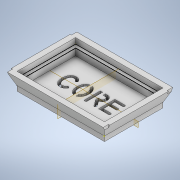
# Autodesk Inventor part: Rack holder Kinpen V2
Saved by Autodesk Inventor 2022 (Build 260153000, 153)
## iProperties
Created: 2021-05-21
Part Number: Rack holder Kinpen V2
Material: Generic
Document SubType Name: Modeling
Designer: Olivi
Density: 1 g/cm^3
Appearance: Default
Author: Olivi
Autodesk Inventor part; units mm, degrees
ref_plane "YZ Plane" through (0, 0, 0) normal (1, 0, 0) x (0, 1, 0)
ref_plane "XZ Plane" through (0, 0, 0) normal (0, 1, 0) x (-1, 0, 0)
ref_plane "XY Plane" through (0, 0, 0) normal (0, 0, 1) x (1, 0, 0)
sketch "Sketch1" plane through (0, 0, 0) normal (0, 1, 0) x (-1, 0, 0)
  line L0 (0, 0) -> (0, -85.5)
  line L1 (0, -85.5) -> (127.8, -85.5)
  line L2 (127.8, -85.5) -> (127.8, 0)
  line L3 (127.8, 0) -> (0, 0)
  dimension "d0" = 85.5
  dimension "d1" = 127.8
  constraints: 8 end point, 3 perpendicular, 1 vertical
  measures "d0" distance of L0.start L0.end
  measures "d1" distance of L0.end L1.end
extrude "Extrusion2" add sketch "Sketch1" along normal blind 7
sketch "Sketch3" plane through (0, 7, 0) normal (0, 1, 0) x (1, 0, 0)
  point P0 (0, 0)
sketch "Sketch5" plane through (0, 7, 0) normal (0, 1, 0) x (1, 0, 0)
  line L0 (-127.8, 0) -> (0, 0) projected
  line L1 (-127.8, 0) -> (0, 0)
  line L2 (0, 0) -> (0, 85.5) projected
  line L3 (0, 0) -> (0, 85.5)
  line L4 (0, 85.5) -> (-127.8, 85.5) projected
  line L5 (0, 85.5) -> (-127.8, 85.5)
  line L6 (-127.8, 85.5) -> (-127.8, 0)
  line L7 (-122.8, 80.5) -> (-5, 80.5)
  line L8 (-5, 80.5) -> (-5, 4.1226)
  line L9 (-5, 4.1226) -> (-122.8, 4.1226)
  line L10 (-122.8, 4.1226) -> (-122.8, 80.5)
  line L11 (-127.8, 85.5) -> (-127.8, 0) projected
  dimension "d44" = 5
  dimension "d45" = 5
  dimension "d46" = 5
  constraints: 16 end point, 5 perpendicular, 3 equal length
  measures "d44" distance between parallel lines of L2 L8
  measures "d45" distance between parallel lines of L6 L10
  measures "d46" distance between parallel lines of L4 L7
extrude "Extrusion4" add sketch "Sketch5" along normal blind 10
sketch "Sketch9" plane through (0, 17, 0) normal (0, 1, 0) x (1, 0, 0)
  line L0 (-127.8, 85.5) -> (-127.8, 0) projected
  line L1 (-127.8, 0) -> (-127.8, 85.5)
  line L2 (-127.8, 85.5) -> (0, 85.5)
  line L3 (0, 85.5) -> (0, 0)
  line L4 (0, 0) -> (-127.8, 0)
  line L5 (-122.8, 4.1226) -> (-5, 4.1226) projected
  line L6 (-5, 80.5) -> (-122.8, 80.5) projected
  line L7 (-122.8, 4.1226) -> (-122.8, 80.5)
  line L8 (-122.8, 80.5) -> (-5, 80.5)
  line L9 (-5, 80.5) -> (-5, 4.1226)
  line L10 (-5, 4.1226) -> (-122.8, 4.1226)
  point P0 (0, 0)
  constraints: 16 end point, 5 equal length, 3 perpendicular
ref_plane "Work Plane4" through (-63.9, 0, 0) normal (1, 0, 0) x (0, 0, -1)
sketch "Sketch21" plane through (-63.9, 0, 0) normal (1, 0, 0) x (0, 0, -1)
  line L0 (0, 0) -> (0, 17) projected
  line L1 (0, 7.0438) -> (0, 25.0438)
  line L2 (0, 25.0438) -> (-8, 25.0438)
  line L3 (-8, 25.0438) -> (0, 7.0438)
  line L4 (85.5, 0) -> (85.5, 17) projected
  line L5 (85.5, 7.0438) -> (85.5, 25.0438)
  line L6 (85.5, 25.0438) -> (93.5, 25.0438)
  line L7 (93.5, 25.0438) -> (85.5, 7.0438)
  dimension "d99" = 18
  dimension "d100" = 8
  dimension "d101" = 18
  dimension "d102" = 8
  constraints: 12 end point, 2 collinear, 2 perpendicular, 2 point on line
  measures "d99" distance of L1.start L1.end
  measures "d100" distance of L1.end L2.end
  measures "d101" distance of L5.start L5.end
  measures "d102" distance of L5.end L6.end
extrude "Extrusion7" add sketch "Sketch21" along normal mid plane 140
ref_plane "Work Plane5" through (-127.8, 0, -42.7) normal (0, 0, 1) x (1, 0, 0)
sketch "Sketch22" plane through (-127.8, 0, -42.7) normal (0, 0, 1) x (1, 0, 0)
  line L0 (127.8, 7.0438) -> (133.9, 7.0438) projected
  line L1 (127.8, 7.0438) -> (127.8, 25.0438)
  line L2 (133.9, 25.0438) -> (-6.1, 25.0438) projected
  line L3 (127.8, 25.0438) -> (135.8, 25.0438)
  line L4 (135.8, 25.0438) -> (127.8, 7.0438)
  line L5 (0, 0) -> (0, 7.0438) projected
  line L6 (0, 7.0438) -> (0, 25.0438)
  line L7 (0, 25.0438) -> (-8, 25.0438)
  line L8 (-6.1, 7.0438) -> (0, 7.0438) projected
  line L9 (-8, 25.0438) -> (0, 7.0438)
  point P0 (127.8, 0)
  dimension "d106" = 8
  dimension "d107" = 8
  constraints: 12 end point, 3 point on line, 2 perpendicular, 1 vertical
  measures "d106" distance of L1.end L3.end
  measures "d107" distance of L6.end L7.end
extrude "Extrusion8" add sketch "Sketch22" along normal mid plane 86
sketch "Sketch24" plane through (-127.8, 0, 0) normal (0, 0, 1) x (1, 0, 0)
  line L0 (-6.1, 7.0438) -> (-6.1, 25.0438) projected
  line L1 (0, 7.0438) -> (127.8, 7.0438) projected
  line L2 (-6.1, 20.9849) -> (0, 7.0438)
  line L3 (0, 7.0438) -> (-6.1, 7.0438)
  line L4 (-6.1, 7.0438) -> (-6.1, 20.9849)
  line L5 (127.8, 7.0438) -> (133.9, 7.0438) projected
  line L6 (133.9, 7.0438) -> (133.9, 20.7688) projected
  line L7 (127.8, 7.0438) -> (133.9, 20.7688)
  line L8 (133.9, 20.7688) -> (133.9, 7.0438)
  line L9 (133.9, 7.0438) -> (127.8, 7.0438)
  point P0 (127.8, 0)
  constraints: 12 end point, 2 collinear, 2 perpendicular, 1 point on line
extrude "Extrusion9" cut sketch "Sketch24" along normal blind 86
sketch "Sketch25" plane through (0, 0, -85.5) normal (0, 0, -1) x (-1, 0, 0)
  line L0 (-6.1, 20.7688) -> (0, 7.0438) projected
  line L1 (0, 7.0438) -> (-6.1, 20.7688)
  line L2 (-6.1, 20.7688) -> (-6.1, 7.0438)
  line L3 (-6.1, 7.0438) -> (0, 7.0438)
  line L4 (127.8, 7.0438) -> (133.9, 20.7688) projected
  line L5 (127.8, 7.0438) -> (133.9, 20.7688)
  line L6 (133.9, 7.0438) -> (133.9, 20.7688) projected
  line L7 (133.9, 20.7688) -> (133.9, 7.0438)
  line L8 (127.8, 7.0438) -> (0, 7.0438) projected
  line L9 (133.9, 7.0438) -> (127.8, 7.0438)
  point P0 (0, 0)
  constraints: 12 end point, 3 collinear, 2 perpendicular, 1 point on line, 1 vertical
extrude "Extrusion10" cut sketch "Sketch25" along normal blind 86
sketch "Sketch26" plane through (0, 7, 0) normal (0, 1, 0) x (1, 0, 0)
  line L0 (-106.3, 54.404) -> (-23.0142, 54.404) construction
  line L1 (-23.0142, 54.404) -> (-23.0142, 29.6305) construction
  line L2 (-23.0142, 29.6305) -> (-106.3, 29.6305) construction
  line L3 (-106.3, 29.6305) -> (-106.3, 54.404) construction
  line L4 (-122.8, 80.5) -> (-5, 80.5) projected
  line L5 (-5, 4.1226) -> (-122.8, 4.1226) projected
  line L6 (-122.8, 4.1226) -> (-122.8, 80.5) projected
  spline S0 degree 2 poles (-87.6379, 33.5693) (-89.4205, 31.3781) (-92.8187, 29.6883) (-95.2142, 29.6883) knots 0 0 0 1 2 2 2
  spline S1 degree 2 poles (-95.2142, 29.6883) (-99.2994, 29.6883) (-101.8805, 33.1422) knots 0 0 0 1 1 1
  spline S2 degree 2 poles (-101.8805, 33.1422) (-104.5359, 36.6332) (-104.5359, 42.2783) knots 0 0 0 1 1 1
  spline S3 degree 2 poles (-104.5359, 42.2783) (-104.5359, 48.5175) (-101.5463, 51.7857) knots 0 0 0 1 1 1
  spline S4 degree 2 poles (-101.5463, 51.7857) (-99.1508, 54.404) (-95.697, 54.404) knots 0 0 0 1 1 1
  spline S5 degree 2 poles (-95.697, 54.404) (-93.0044, 54.404) (-91.4446, 53.6055) knots 0 0 0 1 1 1
  spline S6 degree 2 poles (-91.4446, 53.6055) (-89.7177, 52.7142) (-88.5107, 50.5045) knots 0 0 0 1 1 1
  spline S7 degree 2 poles (-88.5107, 50.5045) (-88.2507, 50.0402) (-88.2507, 49.6131) knots 0 0 0 1 1 1
  spline S8 degree 2 poles (-88.2507, 49.6131) (-88.2507, 48.8704) (-89.3648, 47.8491) (-90.0519, 47.8491) knots 0 0 0 1 2 2 2
  spline S9 degree 2 poles (-90.0519, 47.8491) (-91.0175, 47.8491) (-91.5746, 48.8889) knots 0 0 0 1 1 1
  spline S10 degree 2 poles (-91.5746, 48.8889) (-92.2059, 49.9659) (-93.283, 50.4302) knots 0 0 0 1 1 1
  spline S11 degree 2 poles (-93.283, 50.4302) (-94.1, 50.8201) (-95.7155, 50.8201) knots 0 0 0 1 1 1
  spline S12 degree 2 poles (-95.7155, 50.8201) (-97.8139, 50.8201) (-99.2623, 48.9446) knots 0 0 0 1 1 1
  spline S13 degree 2 poles (-99.2623, 48.9446) (-101.0449, 46.6792) (-101.0449, 42.2783) knots 0 0 0 1 1 1
  spline S14 degree 2 poles (-101.0449, 42.2783) (-101.0449, 38.2302) (-97.6839, 33.2722) (-95.1584, 33.2722) knots 0 0 0 1 2 2 2
  spline S15 degree 2 poles (-95.1584, 33.2722) (-92.4288, 33.2722) (-90.3676, 35.8719) knots 0 0 0 1 1 1
  spline S16 degree 2 poles (-90.3676, 35.8719) (-89.8476, 36.5032) (-89.0492, 36.5032) knots 0 0 0 1 1 1
  spline S17 degree 2 poles (-89.0492, 36.5032) (-88.3621, 36.5032) (-87.2108, 35.4077) (-87.2108, 34.6835) knots 0 0 0 1 2 2 2
  spline S18 degree 2 poles (-87.2108, 34.6835) (-87.2108, 34.0892) (-87.6379, 33.5693) knots 0 0 0 1 1 1
  spline S19 degree 2 poles (-64.3335, 41.944) (-64.3335, 37.0417) (-66.6361, 33.8478) knots 0 0 0 1 1 1
  spline S20 degree 2 poles (-66.6361, 33.8478) (-69.3286, 29.6883) (-73.4696, 29.6883) knots 0 0 0 1 1 1
  spline S21 degree 2 poles (-73.4696, 29.6883) (-77.6291, 29.6883) (-80.2845, 33.5322) knots 0 0 0 1 1 1
  spline S22 degree 2 poles (-80.2845, 33.5322) (-82.7542, 37.0603) (-82.7542, 41.944) knots 0 0 0 1 1 1
  spline S23 degree 2 poles (-82.7542, 41.944) (-82.7542, 46.8277) (-80.433, 50.4116) knots 0 0 0 1 1 1
  spline S24 degree 2 poles (-80.433, 50.4116) (-77.8705, 54.404) (-73.8595, 54.404) knots 0 0 0 1 1 1
  spline S25 degree 2 poles (-73.8595, 54.404) (-69.57, 54.404) (-66.8032, 50.4302) knots 0 0 0 1 1 1
  spline S26 degree 2 poles (-66.8032, 50.4302) (-64.3335, 46.8277) (-64.3335, 41.944) knots 0 0 0 1 1 1
  spline S27 degree 2 poles (-67.8616, 41.944) (-67.8616, 45.5093) (-69.4215, 48.1833) knots 0 0 0 1 1 1
  spline S28 degree 2 poles (-69.4215, 48.1833) (-71.0556, 50.8201) (-73.8595, 50.8201) knots 0 0 0 1 1 1
  spline S29 degree 2 poles (-73.8595, 50.8201) (-76.4406, 50.8201) (-78.0376, 47.8862) knots 0 0 0 1 1 1
  spline S30 degree 2 poles (-78.0376, 47.8862) (-79.226, 45.6022) (-79.226, 41.944) knots 0 0 0 1 1 1
  spline S31 degree 2 poles (-79.226, 41.944) (-79.226, 38.3602) (-78.1304, 36.1133) knots 0 0 0 1 1 1
  spline S32 degree 2 poles (-78.1304, 36.1133) (-76.1807, 33.2722) (-73.4696, 33.2722) knots 0 0 0 1 1 1
  spline S33 degree 2 poles (-73.4696, 33.2722) (-70.7956, 33.2722) (-69.1244, 36.1133) knots 0 0 0 1 1 1
  spline S34 degree 2 poles (-69.1244, 36.1133) (-67.8616, 38.323) (-67.8616, 41.944) knots 0 0 0 1 1 1
  spline S35 degree 2 poles (-42.9417, 47.032) (-42.9417, 43.281) (-45.9871, 41.2941) knots 0 0 0 1 1 1
  spline S36 degree 2 poles (-45.9871, 41.2941) (-47.0641, 40.1242) (-48.7353, 40.1242) knots 0 0 0 1 1 1
  line L7 (-48.7353, 40.1242) -> (-43.2945, 32.7708)
  spline S37 degree 2 poles (-43.2945, 32.7708) (-42.9417, 32.2323) (-42.9417, 31.6938) knots 0 0 0 1 1 1
  spline S38 degree 2 poles (-42.9417, 31.6938) (-42.9417, 30.951) (-44.0373, 29.8554) (-44.7429, 29.8554) knots 0 0 0 1 2 2 2
  spline S39 degree 2 poles (-44.7429, 29.8554) (-45.5785, 29.8554) (-46.117, 30.6725) knots 0 0 0 1 1 1
  line L8 (-46.117, 30.6725) -> (-52.7834, 40.1242)
  line L9 (-52.7834, 40.1242) -> (-56.7572, 40.1242)
  line L10 (-56.7572, 40.1242) -> (-56.7572, 31.6938)
  spline S40 degree 2 poles (-56.7572, 31.6938) (-56.7572, 29.8554) (-58.5213, 29.8554) knots 0 0 0 1 1 1
  spline S41 degree 2 poles (-58.5213, 29.8554) (-60.2854, 29.8554) (-60.2854, 31.6938) knots 0 0 0 1 1 1
  line L11 (-60.2854, 31.6938) -> (-60.2854, 54.1626)
  line L12 (-60.2854, 54.1626) -> (-49.9795, 54.1626)
  spline S42 degree 2 poles (-49.9795, 54.1626) (-47.1198, 54.1626) (-45.0957, 52.3242) knots 0 0 0 1 1 1
  spline S43 degree 2 poles (-45.0957, 52.3242) (-42.9417, 50.2816) (-42.9417, 47.032) knots 0 0 0 1 1 1
  spline S44 degree 2 poles (-46.4327, 47.032) (-46.4327, 48.7032) (-47.3426, 49.6131) knots 0 0 0 1 1 1
  spline S45 degree 2 poles (-47.3426, 49.6131) (-48.4939, 50.6159) (-49.9795, 50.6159) knots 0 0 0 1 1 1
  line L13 (-49.9795, 50.6159) -> (-56.7572, 50.6159)
  line L14 (-56.7572, 50.6159) -> (-56.7572, 43.7081)
  line L15 (-56.7572, 43.7081) -> (-48.7353, 43.7081)
  spline S46 degree 2 poles (-48.7353, 43.7081) (-48.1225, 43.7081) (-47.4169, 44.3395) knots 0 0 0 1 1 1
  spline S47 degree 2 poles (-47.4169, 44.3395) (-46.4327, 45.2494) (-46.4327, 47.032) knots 0 0 0 1 1 1
  line L16 (-24.4467, 30.1711) -> (-38.8936, 30.1711)
  line L17 (-38.8936, 30.1711) -> (-38.8936, 54.1812)
  line L18 (-38.8936, 54.1812) -> (-24.4467, 54.1812)
  spline S48 degree 2 poles (-24.4467, 54.1812) (-22.6826, 54.1812) (-22.6826, 52.3985) knots 0 0 0 1 1 1
  spline S49 degree 2 poles (-22.6826, 52.3985) (-22.6826, 50.5973) (-24.4467, 50.5973) knots 0 0 0 1 1 1
  line L19 (-24.4467, 50.5973) -> (-35.4026, 50.5973)
  line L20 (-35.4026, 50.5973) -> (-35.4026, 45.0822)
  line L21 (-35.4026, 45.0822) -> (-25.1338, 45.0822)
  spline S50 degree 2 poles (-25.1338, 45.0822) (-23.3697, 45.0822) (-23.3697, 43.2996) knots 0 0 0 1 1 1
  spline S51 degree 2 poles (-23.3697, 43.2996) (-23.3697, 41.4984) (-25.1338, 41.4984) knots 0 0 0 1 1 1
  line L22 (-25.1338, 41.4984) -> (-35.4026, 41.4984)
  line L23 (-35.4026, 41.4984) -> (-35.4026, 33.755)
  line L24 (-35.4026, 33.755) -> (-24.4467, 33.755)
  spline S52 degree 2 poles (-24.4467, 33.755) (-22.6826, 33.755) (-22.6826, 31.9723) knots 0 0 0 1 1 1
  spline S53 degree 2 poles (-22.6826, 31.9723) (-22.6826, 30.1711) (-24.4467, 30.1711) knots 0 0 0 1 1 1
  point P0 (0, 0)
  dimension "d114" = 26.096
  dimension "d117" = 16.5
  constraints: 2 other
  measures "d114" distance between parallel lines of L4 L0
  measures "d117" distance between parallel lines of L6 L3
extrude "Extrusion11" cut sketch "Sketch26" against normal blind 8
sketch "Sketch28" plane through (0, 7, 0) normal (0, 1, 0) x (1, 0, 0)
  line L0 (-56.7572, 40.1242) -> (-56.7572, 31.6938) projected
  line L1 (-60.2854, 54.1626) -> (-49.9795, 54.1626) projected
  line L2 (-56.7572, 38.6928) -> (-52.7832, 38.6928)
  line L3 (-52.7832, 38.6928) -> (-52.7832, 54.1626)
  line L4 (-52.7832, 54.1626) -> (-56.7572, 54.1626)
  line L5 (-56.7572, 54.1626) -> (-56.7572, 38.6928)
  line L6 (-71.4826, 35.0297) -> (-75.4566, 35.0297)
  line L7 (-75.4566, 35.0297) -> (-75.4566, 28.7344)
  line L8 (-75.4566, 28.7344) -> (-71.4826, 28.7344)
  line L9 (-71.4826, 28.7344) -> (-71.4826, 35.0297)
  line L10 (-71.4826, 49.1525) -> (-75.4566, 49.1525)
  line L11 (-75.4566, 49.1525) -> (-75.4566, 55.6725)
  line L12 (-75.4566, 55.6725) -> (-71.4826, 55.6725)
  line L13 (-71.4826, 55.6725) -> (-71.4826, 49.1525)
  point P0 (0, 0)
  point P1 (-73.4696, 33.2722)
  dimension "d120" = 3.974
  dimension "d121" = 1.987
  constraints: 24 end point, 7 parallel, 3 horizontal, 3 perpendicular, 2 point on line
  measures "d120" distance of L2.start L2.end
  measures "d121" distance from line of L9 point (-73.47, 33.272)
extrude "Extrusion12" add sketch "Sketch28" against normal blind 8
body "Solid2"
